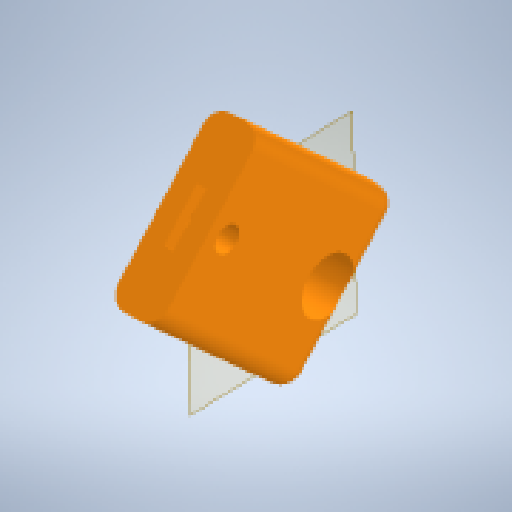
# Autodesk Inventor part: хвост
Saved by Autodesk Inventor 2024.2 (Build 282272000, 272)
## iProperties
Created: 2026-04-03
Part Number: хвост
Material: Типовые
Document SubType Name: Modeling
Designer: katya_notebook
Density: 1 g/cm^3
Appearance: Оранжевый
Author: katya_notebook
Autodesk Inventor part; units mm, degrees
ref_plane "YZ Plane" through (0, 0, 0) normal (1, 0, 0) x (0, 1, 0)
ref_plane "XZ Plane" through (0, 0, 0) normal (0, 1, 0) x (-1, 0, 0)
ref_plane "XY Plane" through (0, 0, 0) normal (0, 0, 1) x (1, 0, 0)
ref_plane "РабПлоскость1" through (-185.8888, -38.5334, 331.0061) normal (0.9999756, 0.0023998, -0.0065586) x (-0.0066118, 0.0228778, -0.9997164)
sketch "Эскиз9" plane through (-185.8888, -38.5334, 331.0061) normal (0.9999756, 0.0023998, -0.0065586) x (-0.0066118, 0.0228778, -0.9997164)
  circle A0 centre (-0.0036, 0) radius 3.25 projected
  line L0 (7.5744, -20.841) -> (-21.2183, 6.4584)
  line L1 (-21.2183, 6.4584) -> (-7.5816, 20.841)
  line L2 (-7.5816, 20.841) -> (21.2112, -6.4584)
  line L3 (21.2112, -6.4584) -> (7.5744, -20.841)
  line L4 (7.5744, -20.841) -> (-7.5816, 20.841) construction
  line L5 (-21.2183, 6.4584) -> (21.2112, -6.4584) construction
  line L6 (9.6794, 4.4753) -> (-3.9573, -9.9074)
  point P0 (330.5647, 30.5274)
  constraints: 14 end point, 3 parallel, 2 midpoint, 2 point on line, 1 perpendicular
extrude "Выдавливание4" add sketch "Эскиз9" along normal blind 6 contours L0 L1 L2 L6
fillet "Сопряжение2" radius 2 8 edges at (-182.8404, -48.5216, 334.7158) (-179.8019, -40.5311, 343.5115) (-185.8017, -40.5455, 343.5509) (-182.963, -33.8307, 321.4122) (-179.9244, -25.8402, 330.2079) (-185.9242, -25.8546, 330.2473) (-185.9016, -41.1833, 328.0837) (-179.9018, -41.1689, 328.0443)
sketch "Эскиз11" plane through (-185.7754, -31.0798, 351.0238) normal (0.0032506, 0.6712535, 0.7412207) x (0.9999756, 0.0023998, -0.0065586)
  line L0 (0, 17.8197) -> (6, -2)
  line L1 (6, 17.8197) -> (0, -2)
  line L2 (2.4, 11.0099) -> (3.6, 11.0099)
  line L3 (3.6, 11.0099) -> (3.6, 4.8099)
  line L4 (3.6, 4.8099) -> (2.4, 4.8099)
  line L5 (2.4, 4.8099) -> (2.4, 11.0099)
  line L6 (2.4, 11.0099) -> (3.6, 4.8099) construction
  line L7 (3.6, 11.0099) -> (2.4, 4.8099) construction
  point P0 (188.1477, 257.5062)
  point P1 (3, 7.9099)
  dimension "d31" = 1.2
  dimension "d32" = 6.2
  constraints: 16 end point, 3 midpoint, 2 parallel, 1 horizontal, 1 perpendicular, 2 other
  measures "d31" distance of L3.end L4.end
  measures "d32" distance of L2.end L3.end
extrude "Выдавливание6" cut sketch "Эскиз11" against normal blind 6
sketch "Эскиз12" plane through (-179.889, -38.519, 330.9668) normal (0.9999756, 0.0023998, -0.0065586) x (-0.0066118, 0.0228778, -0.9997164)
  line L0 (-16.5329, 11.4001) -> (-12.267, 15.8993) projected
  line L1 (-16.5329, 11.4001) -> (-12.1788, 7.2719) projected
  line L2 (-12.1788, 7.2719) -> (-7.913, 11.7711) projected
  line L3 (-12.267, 15.8993) -> (-7.913, 11.7711) projected
  line L4 (-12.1788, 7.2719) -> (-12.267, 15.8993)
  line L5 (-16.5329, 11.4001) -> (-7.913, 11.7711)
  circle A0 centre (-12.2229, 11.5856) radius 1.5
  point P0 (330.5647, 30.5274)
  dimension "d35" = 3
  constraints: 4 end point, 1 centre point, 1 midpoint
  measures "d35" diameter of A0
extrude "Выдавливание7" cut sketch "Эскиз12" against normal blind 6 contours A0 L4 L5 | L5 L4 A0 | A0 L5 L4 | L4 L5 A0
